Autodesk Fusion 360 part; units mm, degrees
(part 2 of 2)
sketch "スケッチ7 (3)" plane through (0, 0, 10.11) normal (0, 0, 1) x (1, 0, 0) in component "Robot V1 - B Front Cover"
  arc A0 (9.5, 66) -> (7.5, 68) centre (7.5, 66) ccw
  arc A1 (7.5, 56) -> (9.5, 58) centre (7.5, 58) ccw
  arc A2 (-16.5, 58) -> (-14.5, 56) centre (-14.5, 58) ccw
  arc A3 (-14.5, 68) -> (-16.5, 66) centre (-14.5, 66) ccw
  line L0 (-14.5, 68) -> (7.5, 68)
  line L1 (9.5, 66) -> (9.5, 58)
  line L2 (7.5, 56) -> (-14.5, 56)
  line L3 (-16.5, 58) -> (-16.5, 66)
  line L4 (7.5, 66) -> (-14.5, 58) construction
  point P0 (-3.5, 62)
  dimension "d1668" = 22
  dimension "d1669" = 8
  dimension "d1670" = 2
  dimension "d1671" = 3.5
  dimension "d1672" = 62
  constraint horizontal L0
  constraint horizontal L2
  constraint vertical L3
  constraint vertical L1
  constraint tangent A0 L0
  constraint tangent A0 L1
  constraint tangent A1 L1
  constraint tangent A1 L2
  constraint tangent A2 L2
  constraint tangent A2 L3
  constraint tangent A3 L3
  constraint tangent A3 L0
  constraint equal A0 A1
  constraint equal A0 A2
  constraint equal A0 A3
  constraint midpoint L4 P0
  measures "d1668" horizontal distance of A0.end A3.start
  measures "d1669" vertical distance of A0.start A1.end
  measures "d1670" radius of A0
  measures "d1671" horizontal distance of origin P0
  measures "d1672" vertical distance of origin P0
extrude "B07 Forehead opening" cut sketch "スケッチ7 (3)" against normal blind 2.4 bodies 18 in component "Robot V1 - B Front Cover"
sketch "スケッチ8 (3)" plane through (0, 0, 10.11) normal (0, 0, 1) x (1, 0, 0) in component "Robot V1 - B Front Cover"
  circle A0 centre (0, -59.97) radius 7
  dimension "d1675" = 59.97
  dimension "d1676" = 14
  constraint vertical origin A0.centre
  measures "d1675" vertical distance of origin A0.centre
  measures "d1676" diameter of A0
extrude "B08 Home access" cut sketch "スケッチ8 (3)" against normal blind 2.4 bodies 18 in component "Robot V1 - B Front Cover"
sketch "スケッチ9 (3)" plane through (0, 0, 10.11) normal (0, 0, 1) x (1, 0, 0) in component "Robot V1 - B Front Cover"
  line L0 (12, 16.1) -> (-12, 16.1)
  line L1 (-12, 16.1) -> (-12, 14.9)
  line L2 (-12, 14.9) -> (12, 14.9)
  line L3 (12, 14.9) -> (12, 16.1)
  line L4 (12, 16.1) -> (-12, 14.9) construction
  point P0 (0, 15.5)
  dimension "d1679" = 15.5
  dimension "d1680" = 24
  dimension "d1681" = 1.2
  constraint horizontal L0
  constraint vertical L1
  constraint horizontal L2
  constraint vertical L3
  constraint midpoint L4 P0
  constraint vertical origin P0
  measures "d1679" vertical distance of origin P0
  measures "d1680" horizontal distance of L0.start L0.end
  measures "d1681" vertical distance of L0.end L1.end
extrude "B09 Shallow mouth groove" cut sketch "スケッチ9 (3)" against normal blind 0.6 bodies 18 in component "Robot V1 - B Front Cover"
sketch "スケッチ19 (2)" plane through (0, 0, 7.71) normal (0, 0, 1) x (1, 0, 0) in component "Robot V1 - A Holder and Stand"
  circle A0 centre (-40, 62) radius 1.7
  dimension "d1684" = 40
  dimension "d1685" = 62
  dimension "d1686" = 3.4
  measures "d1684" horizontal distance of origin A0.centre
  measures "d1685" vertical distance of origin A0.centre
  measures "d1686" diameter of A0
extrude "A20 TL bolt hole" cut sketch "スケッチ19 (2)" against normal blind 10.61 bodies 17 in component "Robot V1 - A Holder and Stand"
sketch "スケッチ20" plane through (0, 0, 7.71) normal (0, 0, 1) x (1, 0, 0) in component "Robot V1 - A Holder and Stand"
  circle A0 centre (40, 62) radius 1.7
  dimension "d1689" = 40
  dimension "d1690" = 62
  dimension "d1691" = 3.4
  measures "d1689" horizontal distance of origin A0.centre
  measures "d1690" vertical distance of origin A0.centre
  measures "d1691" diameter of A0
extrude "A20 TR bolt hole" cut sketch "スケッチ20" against normal blind 10.61 bodies 17 in component "Robot V1 - A Holder and Stand"
sketch "スケッチ21" plane through (0, 0, 7.71) normal (0, 0, 1) x (1, 0, 0) in component "Robot V1 - A Holder and Stand"
  circle A0 centre (-37, -62) radius 1.7
  dimension "d1694" = 37
  dimension "d1695" = 62
  dimension "d1696" = 3.4
  measures "d1694" horizontal distance of origin A0.centre
  measures "d1695" vertical distance of origin A0.centre
  measures "d1696" diameter of A0
extrude "A20 BL bolt hole" cut sketch "スケッチ21" against normal blind 10.61 bodies 17 in component "Robot V1 - A Holder and Stand"
sketch "スケッチ22" plane through (0, 0, 7.71) normal (0, 0, 1) x (1, 0, 0) in component "Robot V1 - A Holder and Stand"
  circle A0 centre (37, -62) radius 1.7
  dimension "d1699" = 37
  dimension "d1700" = 62
  dimension "d1701" = 3.4
  measures "d1699" horizontal distance of origin A0.centre
  measures "d1700" vertical distance of origin A0.centre
  measures "d1701" diameter of A0
extrude "A20 BR bolt hole" cut sketch "スケッチ22" against normal blind 10.61 bodies 17 in component "Robot V1 - A Holder and Stand"
sketch "スケッチ10 (3)" plane through (0, 0, 10.11) normal (0, 0, 1) x (1, 0, 0) in component "Robot V1 - B Front Cover"
  circle A0 centre (-40, 62) radius 1.7
  dimension "d1704" = 40
  dimension "d1705" = 62
  dimension "d1706" = 3.4
  measures "d1704" horizontal distance of origin A0.centre
  measures "d1705" vertical distance of origin A0.centre
  measures "d1706" diameter of A0
extrude "B20 TL bolt hole" cut sketch "スケッチ10 (3)" against normal blind 2.4 bodies 18 in component "Robot V1 - B Front Cover"
sketch "スケッチ11 (3)" plane through (0, 0, 10.11) normal (0, 0, 1) x (1, 0, 0) in component "Robot V1 - B Front Cover"
  circle A0 centre (40, 62) radius 1.7
  dimension "d1709" = 40
  dimension "d1710" = 62
  dimension "d1711" = 3.4
  measures "d1709" horizontal distance of origin A0.centre
  measures "d1710" vertical distance of origin A0.centre
  measures "d1711" diameter of A0
extrude "B20 TR bolt hole" cut sketch "スケッチ11 (3)" against normal blind 2.4 bodies 18 in component "Robot V1 - B Front Cover"
sketch "スケッチ12 (3)" plane through (0, 0, 10.11) normal (0, 0, 1) x (1, 0, 0) in component "Robot V1 - B Front Cover"
  circle A0 centre (-37, -62) radius 1.7
  dimension "d1714" = 37
  dimension "d1715" = 62
  dimension "d1716" = 3.4
  measures "d1714" horizontal distance of origin A0.centre
  measures "d1715" vertical distance of origin A0.centre
  measures "d1716" diameter of A0
extrude "B20 BL bolt hole" cut sketch "スケッチ12 (3)" against normal blind 2.4 bodies 18 in component "Robot V1 - B Front Cover"
sketch "スケッチ13 (3)" plane through (0, 0, 10.11) normal (0, 0, 1) x (1, 0, 0) in component "Robot V1 - B Front Cover"
  circle A0 centre (37, -62) radius 1.7
  dimension "d1719" = 37
  dimension "d1720" = 62
  dimension "d1721" = 3.4
  measures "d1719" horizontal distance of origin A0.centre
  measures "d1720" vertical distance of origin A0.centre
  measures "d1721" diameter of A0
extrude "B20 BR bolt hole" cut sketch "スケッチ13 (3)" against normal blind 2.4 bodies 18 in component "Robot V1 - B Front Cover"
component "iPhone SE 3 - Parametric Drawing Model" placed x (1, 0, 0) y (0, 1, 0) z (0, 0, 1) at (0, 0, 0)
component "Robot V1 - A Holder and Stand" placed x (1, 0, 0) y (0, 1, 0) z (0, 0, 1) at (0, 0, 0)
component "Robot V1 - B Front Cover" placed x (1, 0, 0) y (0, 1, 0) z (0, 0, 1) at (0, 0, 0)
equation "SE3_OverallWidth = 67.27 mm" comment "Overall product width"
equation "SE3_OverallHeight = 138.44 mm" comment "Overall product height"
equation "SE3_ProductThickness = 7.31 mm" comment "Nominal product thickness"
equation "SE3_CornerRadius = 9.10 mm" comment "Parameterized plan-view corner radius"
equation "SE3_RearGlassThickness = 0.90 mm" comment "Modeled rear glass thickness"
equation "SE3_FrontGlassThickness = 0.90 mm" comment "Modeled front glass thickness"
equation "SE3_ActiveWidth = 58.50 mm" comment "Front active-area width"
equation "SE3_ActiveHeight = 104.05 mm" comment "Front active-area height"
equation "SE3_ActiveTopOffset = 17.19 mm" comment "Top product datum to active area"
equation "SE3_HomeDiameter = 10.90 mm" comment "Home/Touch ID sensor diameter"
equation "SE3_HomeBottomOffset = 9.25 mm" comment "Bottom datum to Home sensor center"
equation "SE3_ReceiverWidth = 11.87 mm" comment "Receiver width"
equation "SE3_ReceiverHeight = 1.20 mm" comment "Receiver height"
equation "SE3_ReceiverTopOffset = 9.10 mm" comment "Top datum to receiver center"
equation "SE3_FrontCameraDiameter = 3.21 mm" comment "Front camera opening/keepout diameter"
equation "SE3_FrontCameraXFromLeft = 22.99 mm" comment "Left datum to front camera center"
equation "SE3_FrontCameraTopOffset = 9.10 mm" comment "Top datum to front camera center"
equation "SE3_ProximityDiameter = 2.00 mm" comment "Proximity sensor display diameter"
equation "SE3_ProximityXFromLeft = 33.63 mm" comment "Left datum to proximity center"
equation "SE3_ProximityTopOffset = 4.84 mm" comment "Top datum to proximity center"
equation "SE3_ALSDiameter = 2.00 mm" comment "Ambient light sensor display diameter"
equation "SE3_ALSXFromLeft = 37.32 mm" comment "Left datum to ALS center"
equation "SE3_ALSTopOffset = 4.84 mm" comment "Top datum to ALS center"
equation "SE3_RearCameraDiameter = 8.57 mm" comment "Rear camera opening diameter"
equation "SE3_RearMicDiameter = 1.50 mm" comment "Rear microphone diameter"
equation "SE3_RearFlashDiameter = 3.75 mm" comment "Rear flash diameter"
equation "SE3_RearCameraXFromLeft = 10.44 mm" comment "Left datum to rear camera center"
equation "SE3_RearMicXFromLeft = 18.13 mm" comment "Left datum to rear microphone center"
equation "SE3_RearFlashXFromLeft = 22.84 mm" comment "Left datum to rear flash center"
equation "SE3_RearFeatureTopOffset = 15.40 mm" comment "Top datum to rear feature centers"
equation "SE3_CameraBumpHeight = 0.87 mm" comment "Modeled rear camera projection"
equation "SE3_RingTopOffset = 17.56 mm" comment "Top datum to top of ring/silent switch"
equation "SE3_RingLength = 5.61 mm" comment "Ring/silent switch length"
equation "SE3_VolumePlusCenterFromTop = 34.56 mm" comment "Top datum to volume-plus center"
equation "SE3_VolumeMinusCenterFromTop = 47.17 mm" comment "Top datum to volume-minus center"
equation "SE3_ButtonLength = 10.62 mm" comment "Button length: 2 x 5.31"
equation "SE3_ButtonFaceWidth = 1.80 mm" comment "Modeled button width in product-thickness direction"
equation "SE3_RingProjection = 0.42 mm" comment "Ring/silent switch projection"
equation "SE3_ButtonProjection = 0.40 mm" comment "Volume and side-button projection"
equation "SE3_SideButtonCenterFromTop = 34.64 mm" comment "Top datum to side-button center"
equation "SE3_SIMTrayTopOffset = 52.72 mm" comment "Top datum to SIM tray top"
equation "SE3_SIMTrayLength = 15.67 mm" comment "SIM tray length"
equation "SE3_SIMTrayWidth = 2.30 mm" comment "SIM tray visible width"
equation "SE3_BottomHoleDiameter = 1.45 mm" comment "Bottom microphone/speaker hole diameter"
equation "SE3_BottomHoleFirstFromLeft = 10.26 mm" comment "Left datum to first left acoustic hole"
equation "SE3_BottomHolePitch = 2.40 mm" comment "Bottom acoustic-hole pitch: 12.00 / 5"
equation "SE3_BottomRightFirstFromLeft = 45.01 mm" comment "Left datum to first right acoustic hole"
equation "SE3_ScrewDiameter = 1.60 mm" comment "Bottom screw diameter"
equation "SE3_LeftScrewFromLeft = 27.24 mm" comment "Left datum to left screw"
equation "SE3_RightScrewFromLeft = 40.03 mm" comment "Left datum to right screw"
equation "SE3_LightningWidth = 8.70 mm" comment "Lightning opening width: 37.98 - 29.28"
equation "SE3_LightningHeight = 1.60 mm" comment "Modeled Lightning opening height"
equation "SE3_DetailOverlay = 0.02 mm" comment "Visual reference overlay thickness"
equation "d710 = SE3_OverallWidth - 2 * SE3_CornerRadius"
equation "d711 = SE3_OverallHeight - 2 * SE3_CornerRadius"
equation "d712 = SE3_CornerRadius"
equation "d713 = SE3_OverallWidth / 2 - SE3_CornerRadius"
equation "d714 = SE3_OverallHeight / 2 - SE3_CornerRadius"
equation "d715 = SE3_RearGlassThickness"
equation "d717 = SE3_RearGlassThickness"
equation "d719 = SE3_OverallWidth - 2 * SE3_CornerRadius"
equation "d720 = SE3_OverallHeight - 2 * SE3_CornerRadius"
equation "d721 = SE3_CornerRadius"
equation "d722 = SE3_OverallWidth / 2 - SE3_CornerRadius"
equation "d723 = SE3_OverallHeight / 2 - SE3_CornerRadius"
equation "d724 = SE3_ProductThickness - SE3_RearGlassThickness - SE3_FrontGlassThickness"
equation "d726 = SE3_ProductThickness - SE3_FrontGlassThickness"
equation "d728 = SE3_OverallWidth - 2 * SE3_CornerRadius"
equation "d729 = SE3_OverallHeight - 2 * SE3_CornerRadius"
equation "d730 = SE3_CornerRadius"
equation "d731 = SE3_OverallWidth / 2 - SE3_CornerRadius"
equation "d732 = SE3_OverallHeight / 2 - SE3_CornerRadius"
equation "d733 = SE3_FrontGlassThickness"
equation "d735 = SE3_ProductThickness"
equation "d737 = SE3_ActiveWidth - 2 * 0.80 mm"
equation "d738 = SE3_ActiveHeight - 2 * 0.80 mm"
equation "d740 = SE3_ActiveWidth / 2 - 0.80 mm"
equation "d741 = ( SE3_OverallHeight / 2 - SE3_ActiveTopOffset - SE3_ActiveHeight / 2 ) + SE3_ActiveHeight / 2 - 0.80 mm"
equation "d742 = SE3_DetailOverlay"
equation "d744 = SE3_OverallHeight / 2 - SE3_HomeBottomOffset"
equation "d745 = SE3_HomeDiameter"
equation "d746 = SE3_DetailOverlay"
equation "d748 = SE3_OverallWidth / 2 - SE3_FrontCameraXFromLeft"
equation "d749 = SE3_OverallHeight / 2 - SE3_FrontCameraTopOffset"
equation "d750 = SE3_FrontCameraDiameter"
equation "d751 = SE3_DetailOverlay"
equation "d753 = SE3_OverallWidth / 2 - SE3_ProximityXFromLeft"
equation "d754 = SE3_OverallHeight / 2 - SE3_ProximityTopOffset"
equation "d755 = SE3_ProximityDiameter"
equation "d756 = SE3_DetailOverlay"
equation "d758 = SE3_ALSXFromLeft - SE3_OverallWidth / 2"
equation "d759 = SE3_OverallHeight / 2 - SE3_ALSTopOffset"
equation "d760 = SE3_ALSDiameter"
equation "d761 = SE3_DetailOverlay"
equation "d763 = SE3_ReceiverWidth - SE3_ReceiverHeight"
equation "d764 = SE3_ReceiverHeight / 2"
equation "d765 = SE3_OverallHeight / 2 - SE3_ReceiverTopOffset"
equation "d766 = SE3_DetailOverlay"
equation "d768 = SE3_OverallWidth / 2 - SE3_RearCameraXFromLeft"
equation "d769 = SE3_OverallHeight / 2 - SE3_RearFeatureTopOffset"
equation "d770 = SE3_RearCameraDiameter"
equation "d771 = -( SE3_CameraBumpHeight )"
equation "d773 = SE3_OverallWidth / 2 - SE3_RearMicXFromLeft"
equation "d774 = SE3_OverallHeight / 2 - SE3_RearFeatureTopOffset"
equation "d775 = SE3_RearMicDiameter"
equation "d776 = -( SE3_DetailOverlay )"
equation "d778 = SE3_OverallWidth / 2 - SE3_RearFlashXFromLeft"
equation "d779 = SE3_OverallHeight / 2 - SE3_RearFeatureTopOffset"
equation "d780 = SE3_RearFlashDiameter"
equation "d781 = -( SE3_DetailOverlay )"
equation "d783 = -SE3_OverallWidth / 2"
equation "d785 = SE3_OverallWidth / 2"
equation "d787 = SE3_RingLength - SE3_ButtonFaceWidth"
equation "d788 = SE3_ButtonFaceWidth / 2"
equation "d789 = SE3_ProductThickness / 2"
equation "d790 = SE3_OverallHeight / 2 - SE3_RingTopOffset - SE3_RingLength / 2"
equation "d791 = -( SE3_RingProjection )"
equation "d793 = SE3_ButtonLength - SE3_ButtonFaceWidth"
equation "d794 = SE3_ButtonFaceWidth / 2"
equation "d795 = SE3_ProductThickness / 2"
equation "d796 = SE3_OverallHeight / 2 - SE3_VolumePlusCenterFromTop"
equation "d797 = -( SE3_ButtonProjection )"
equation "d799 = SE3_ButtonLength - SE3_ButtonFaceWidth"
equation "d800 = SE3_ButtonFaceWidth / 2"
equation "d801 = SE3_ProductThickness / 2"
equation "d802 = SE3_OverallHeight / 2 - SE3_VolumeMinusCenterFromTop"
equation "d803 = -( SE3_ButtonProjection )"
equation "d805 = SE3_ButtonLength - SE3_ButtonFaceWidth"
equation "d806 = SE3_ButtonFaceWidth / 2"
equation "d807 = SE3_ProductThickness / 2"
equation "d808 = SE3_OverallHeight / 2 - SE3_SideButtonCenterFromTop"
equation "d809 = SE3_ButtonProjection"
equation "d811 = SE3_SIMTrayLength - SE3_SIMTrayWidth"
equation "d812 = SE3_SIMTrayWidth / 2"
equation "d813 = SE3_ProductThickness / 2"
equation "d814 = SE3_OverallHeight / 2 - SE3_SIMTrayTopOffset - SE3_SIMTrayLength / 2"
equation "d815 = -( 0.05 mm )"
equation "d817 = -SE3_OverallHeight / 2"
equation "d819 = SE3_LightningWidth - SE3_LightningHeight"
equation "d820 = SE3_LightningHeight / 2"
equation "d821 = SE3_ProductThickness / 2"
equation "d822 = SE3_OverallWidth / 2 - ( SE3_BottomHoleFirstFromLeft + 0 * SE3_BottomHolePitch )"
equation "d823 = SE3_ProductThickness / 2"
equation "d824 = SE3_BottomHoleDiameter"
equation "d825 = SE3_OverallWidth / 2 - ( SE3_BottomHoleFirstFromLeft + 1 * SE3_BottomHolePitch )"
equation "d826 = SE3_ProductThickness / 2"
equation "d827 = SE3_BottomHoleDiameter"
equation "d828 = SE3_OverallWidth / 2 - ( SE3_BottomHoleFirstFromLeft + 2 * SE3_BottomHolePitch )"
equation "d829 = SE3_ProductThickness / 2"
equation "d830 = SE3_BottomHoleDiameter"
equation "d831 = SE3_OverallWidth / 2 - ( SE3_BottomHoleFirstFromLeft + 3 * SE3_BottomHolePitch )"
equation "d832 = SE3_ProductThickness / 2"
equation "d833 = SE3_BottomHoleDiameter"
equation "d834 = SE3_OverallWidth / 2 - ( SE3_BottomHoleFirstFromLeft + 4 * SE3_BottomHolePitch )"
equation "d835 = SE3_ProductThickness / 2"
equation "d836 = SE3_BottomHoleDiameter"
equation "d837 = SE3_OverallWidth / 2 - ( SE3_BottomHoleFirstFromLeft + 5 * SE3_BottomHolePitch )"
equation "d838 = SE3_ProductThickness / 2"
equation "d839 = SE3_BottomHoleDiameter"
equation "d840 = ( SE3_BottomRightFirstFromLeft + 0 * SE3_BottomHolePitch ) - SE3_OverallWidth / 2"
equation "d841 = SE3_ProductThickness / 2"
equation "d842 = SE3_BottomHoleDiameter"
equation "d843 = ( SE3_BottomRightFirstFromLeft + 1 * SE3_BottomHolePitch ) - SE3_OverallWidth / 2"
equation "d844 = SE3_ProductThickness / 2"
equation "d845 = SE3_BottomHoleDiameter"
equation "d846 = ( SE3_BottomRightFirstFromLeft + 2 * SE3_BottomHolePitch ) - SE3_OverallWidth / 2"
equation "d847 = SE3_ProductThickness / 2"
equation "d848 = SE3_BottomHoleDiameter"
equation "d849 = ( SE3_BottomRightFirstFromLeft + 3 * SE3_BottomHolePitch ) - SE3_OverallWidth / 2"
equation "d850 = SE3_ProductThickness / 2"
equation "d851 = SE3_BottomHoleDiameter"
equation "d852 = ( SE3_BottomRightFirstFromLeft + 4 * SE3_BottomHolePitch ) - SE3_OverallWidth / 2"
equation "d853 = SE3_ProductThickness / 2"
equation "d854 = SE3_BottomHoleDiameter"
equation "d855 = ( SE3_BottomRightFirstFromLeft + 5 * SE3_BottomHolePitch ) - SE3_OverallWidth / 2"
equation "d856 = SE3_ProductThickness / 2"
equation "d857 = SE3_BottomHoleDiameter"
equation "d858 = SE3_OverallWidth / 2 - SE3_LeftScrewFromLeft"
equation "d859 = SE3_ProductThickness / 2"
equation "d860 = SE3_ScrewDiameter"
equation "d861 = SE3_RightScrewFromLeft - SE3_OverallWidth / 2"
equation "d862 = SE3_ProductThickness / 2"
equation "d863 = SE3_ScrewDiameter"
equation "d866 = SE3_ProductThickness / 2"
equation "d868 = SE3_OverallWidth - 2 * SE3_CornerRadius"
equation "d869 = SE3_OverallHeight - 2 * SE3_CornerRadius"
equation "d870 = SE3_CornerRadius"
equation "d871 = SE3_OverallWidth / 2 - SE3_CornerRadius"
equation "d872 = SE3_OverallHeight / 2 - SE3_CornerRadius"
equation "RB_Clearance = 0.4 mm" comment "Phone clearance PER SIDE; test-print before final use"
equation "RB_BackGap = 0.5 mm" comment "Allowance for thin pads between rear glass and tray"
equation "RB_FrontGap = 0.4 mm" comment "Clearance above front glass, excluding screen protector"
equation "RB_Wall = 2.4 mm" comment "Tray side walls"
equation "RB_BackThickness = 2.4 mm" comment "Tray back plate"
equation "RB_CoverThickness = 2.4 mm" comment "Front cover plate"
equation "RB_HeadWidth = 92 mm" comment "Head width, excluding no separate ears"
equation "RB_BodyWidth = 82 mm" comment "Body widened from concept to fit lower M3 screws"
equation "RB_CaseHeight = 148 mm" comment "Cover total height in phone coordinates"
equation "RB_HeadHeight = 60 mm" comment "Top rounded box height"
equation "RB_BodyHeight = 96 mm" comment "Bottom rounded box height; overlaps head"
equation "RB_OuterRadius = 6 mm" comment "Rounded external corners"
equation "RB_EyeWidth = 20 mm" comment "Each eye aperture width"
equation "RB_EyeHeight = 22 mm" comment "Each eye aperture height"
equation "RB_EyeRadius = 8 mm" comment "Eye corner radius, <= half the smaller dimension"
equation "RB_EyeX = 14 mm" comment "Half of eye center spacing"
equation "RB_EyeY = 31 mm" comment "Eye centers above phone center"
equation "RB_BellyWidth = 48 mm" comment "Message window width"
equation "RB_BellyHeight = 28 mm" comment "Message window height"
equation "RB_BellyRadius = 3 mm" comment "Message window corner radius"
equation "RB_BellyY = -3 mm" comment "Message window center Y"
equation "RB_TalkDiameter = 24 mm" comment "Touch aperture at the screen side"
equation "RB_TalkY = -35 mm" comment "Touch aperture center Y"
equation "RB_TouchBevel = 1 mm" comment "45 degree entry bevel; remaining lip is 1.4 mm"
equation "RB_HomeDiameter = 14 mm" comment "Maintenance access, NOT the conversation button"
equation "RB_ForeheadWidth = 26 mm" comment "Camera, receiver, sensors shared forehead opening"
equation "RB_ForeheadHeight = 12 mm" comment "Forehead opening; validate camera field of view"
equation "RB_ForeheadX = -3.5 mm" comment "Forehead opening center X"
equation "RB_ForeheadY = 62 mm" comment "Forehead opening center Y"
equation "RB_MouthWidth = 24 mm" comment "Decorative mouth groove width"
equation "RB_MouthHeight = 1.2 mm" comment "Decorative mouth groove height"
equation "RB_MouthY = 15.5 mm" comment "Decorative mouth center Y"
equation "RB_MouthDepth = 0.6 mm" comment "Blind groove only, no display opening"
equation "RB_ScrewDiameter = 3.4 mm" comment "Through clearance for four M3 bolts and loose nuts"
equation "RB_TopScrewX = 40 mm" comment "Top screw centers +/- X"
equation "RB_TopScrewY = 62 mm" comment "Top screw centers Y"
equation "RB_BottomScrewX = 37 mm" comment "Bottom screw centers +/- X"
equation "RB_BottomScrewY = -62 mm" comment "Bottom screw centers Y"
equation "RB_Tilt = 12 deg" comment "Phone tilt back from vertical on its base"
equation "RB_Lift = 35 mm" comment "Desk to phone lower rear edge; check actual cable"
equation "RB_BaseWidth = 100 mm" comment "Base left-right width"
equation "RB_BaseDepth = 90 mm" comment "Base front-back distance along desk"
equation "RB_BaseFront = 20 mm" comment "Base reach forward from lower rear-edge projection"
equation "RB_BaseThickness = 4 mm" comment "Base thickness normal to desk"
equation "RB_RibThickness = 4 mm" comment "Two rear triangular stand ribs"
equation "RB_RibX = 29 mm" comment "Stand rib center X +/-"
equation "RB_CableWidth = 16 mm" comment "Open-ended cable channel in base"
equation "RB_BottomOpening = 54 mm" comment "Bottom opening clears Lightning and both acoustic rows"
equation "RB_VentWidth = 40 mm" comment "Rear ventilation / finger access width"
equation "RB_VentHeight = 62 mm" comment "Rear ventilation / finger access height"
equation "RB_RearCameraWidth = 26 mm" comment "Rear camera, microphone and flash opening"
equation "RB_RearCameraHeight = 18 mm" comment "Rear camera opening height"
equation "RB_PocketWidth = SE3_OverallWidth + 2 * RB_Clearance" comment "Derived phone pocket width"
equation "RB_PocketHeight = SE3_OverallHeight + 2 * RB_Clearance" comment "Derived phone pocket height"
equation "RB_PocketRadius = SE3_CornerRadius + RB_Clearance" comment "Derived approximate pocket corner radius"
equation "RB_TrayWidth = RB_PocketWidth + 2 * RB_Wall" comment "Derived outer tray width"
equation "RB_TrayHeight = RB_PocketHeight + 2 * RB_Wall" comment "Derived outer tray height"
equation "RB_BackZ = -RB_BackGap - RB_BackThickness" comment "Rear-most tray plane"
equation "RB_CoverZ = SE3_ProductThickness + RB_FrontGap" comment "Cover rear face / tray mating plane"
equation "RB_CoverTopZ = RB_CoverZ + RB_CoverThickness" comment "Cover front face"
equation "RB_DeskY = -SE3_OverallHeight / 2 - RB_Lift / cos(RB_Tilt)" comment "Desk-plane Y intercept at phone Z=0"
equation "d1514 = RB_BackZ"
equation "d1516 = -RB_BackGap"
equation "d1518 = RB_CoverZ"
equation "d1520 = ( RB_HeadWidth ) - 2 * ( RB_OuterRadius )"
equation "d1521 = ( RB_HeadHeight ) - 2 * ( RB_OuterRadius )"
equation "d1522 = RB_OuterRadius"
equation "d1523 = abs(RB_CaseHeight / 2 - RB_HeadHeight / 2)"
equation "d1524 = RB_BackThickness"
equation "d1526 = ( RB_BodyWidth ) - 2 * ( RB_OuterRadius )"
equation "d1527 = ( RB_BodyHeight ) - 2 * ( RB_OuterRadius )"
equation "d1528 = RB_OuterRadius"
equation "d1529 = abs(-RB_CaseHeight / 2 + RB_BodyHeight / 2)"
equation "d1530 = RB_BackThickness"
equation "d1532 = ( RB_TrayWidth ) - 2 * ( RB_PocketRadius + RB_Wall )"
equation "d1533 = ( RB_TrayHeight ) - 2 * ( RB_PocketRadius + RB_Wall )"
equation "d1534 = RB_PocketRadius + RB_Wall"
equation "d1535 = RB_CoverZ + RB_BackGap"
equation "d1537 = abs(-RB_TopScrewX)"
equation "d1538 = abs(RB_TopScrewY)"
equation "d1540 = RB_CoverZ + RB_BackGap"
equation "d1542 = abs(RB_TopScrewX)"
equation "d1543 = abs(RB_TopScrewY)"
equation "d1545 = RB_CoverZ + RB_BackGap"
equation "d1547 = abs(-RB_BottomScrewX)"
equation "d1548 = abs(RB_BottomScrewY)"
equation "d1550 = RB_CoverZ + RB_BackGap"
equation "d1552 = abs(RB_BottomScrewX)"
equation "d1553 = abs(RB_BottomScrewY)"
equation "d1555 = RB_CoverZ + RB_BackGap"
equation "d1557 = ( RB_PocketWidth ) - 2 * ( RB_PocketRadius )"
equation "d1558 = ( RB_PocketHeight ) - 2 * ( RB_PocketRadius )"
equation "d1559 = RB_PocketRadius"
equation "d1560 = -( RB_CoverZ + RB_BackGap )"
equation "d1562 = abs(-RB_TrayWidth / 2)"
equation "d1563 = abs(34 mm)"
equation "d1566 = -( RB_CoverZ + RB_BackGap )"
equation "d1568 = abs(RB_TrayWidth / 2)"
equation "d1569 = abs(34 mm)"
equation "d1572 = -( RB_CoverZ + RB_BackGap )"
equation "d1574 = abs(-RB_CaseHeight / 2)"
equation "d1575 = RB_BottomOpening"
equation "d1577 = -( RB_CoverZ - RB_BackZ )"
equation "d1579 = ( RB_RearCameraWidth ) - 2 * ( 2 mm )"
equation "d1580 = ( RB_RearCameraHeight ) - 2 * ( 2 mm )"
equation "d1582 = abs(-18 mm)"
equation "d1583 = abs(54.5 mm)"
equation "d1584 = -( RB_CoverZ - RB_BackZ )"
equation "d1586 = ( RB_VentWidth ) - 2 * ( 4 mm )"
equation "d1587 = ( RB_VentHeight ) - 2 * ( 4 mm )"
equation "d1589 = abs(-7 mm)"
equation "d1590 = -( RB_CoverZ - RB_BackZ )"
equation "d1592 = -RB_RibX - RB_RibThickness / 2"
equation "d1594 = abs(( -1 ) * ( -RB_BackGap ))"
equation "d1595 = abs(RB_DeskY - ( -RB_BackGap ) * tan(RB_Tilt) + RB_BaseThickness / cos(RB_Tilt) - 0.3 mm)"
equation "d1596 = abs(( -1 ) * ( -( RB_BaseDepth - RB_BaseFront - 4 mm ) * cos(RB_Tilt) ))"
equation "d1597 = abs(RB_DeskY - ( -( RB_BaseDepth - RB_BaseFront - 4 mm ) * cos(RB_Tilt) ) * tan(RB_Tilt) + RB_BaseThickness / cos(RB_Tilt) - 0.3 mm)"
equation "d1598 = RB_RibThickness"
equation "d1600 = RB_RibX - RB_RibThickness / 2"
equation "d1602 = abs(( -1 ) * ( -RB_BackGap ))"
equation "d1603 = abs(RB_DeskY - ( -RB_BackGap ) * tan(RB_Tilt) + RB_BaseThickness / cos(RB_Tilt) - 0.3 mm)"
equation "d1604 = abs(( -1 ) * ( -( RB_BaseDepth - RB_BaseFront - 4 mm ) * cos(RB_Tilt) ))"
equation "d1605 = abs(RB_DeskY - ( -( RB_BaseDepth - RB_BaseFront - 4 mm ) * cos(RB_Tilt) ) * tan(RB_Tilt) + RB_BaseThickness / cos(RB_Tilt) - 0.3 mm)"
equation "d1606 = RB_RibThickness"
equation "d1608 = -RB_BaseWidth / 2"
equation "d1610 = abs(( -1 ) * ( RB_BaseFront * cos(RB_Tilt) ))"
equation "d1611 = abs(RB_DeskY - ( RB_BaseFront * cos(RB_Tilt) ) * tan(RB_Tilt))"
equation "d1612 = abs(( -1 ) * ( -( RB_BaseDepth - RB_BaseFront ) * cos(RB_Tilt) ))"
equation "d1613 = abs(RB_DeskY - ( -( RB_BaseDepth - RB_BaseFront ) * cos(RB_Tilt) ) * tan(RB_Tilt))"
equation "d1614 = abs(( -1 ) * ( ( -( RB_BaseDepth - RB_BaseFront ) * cos(RB_Tilt) ) + RB_BaseThickness * sin(RB_Tilt) ))"
equation "d1615 = abs(RB_DeskY - ( ( -( RB_BaseDepth - RB_BaseFront ) * cos(RB_Tilt) ) + RB_BaseThickness * sin(RB_Tilt) ) * tan(RB_Tilt) + RB_BaseThickness / cos(RB_Tilt))"
equation "d1616 = abs(( -1 ) * ( ( RB_BaseFront * cos(RB_Tilt) ) + RB_BaseThickness * sin(RB_Tilt) ))"
equation "d1617 = abs(RB_DeskY - ( ( RB_BaseFront * cos(RB_Tilt) ) + RB_BaseThickness * sin(RB_Tilt) ) * tan(RB_Tilt) + RB_BaseThickness / cos(RB_Tilt))"
equation "d1618 = RB_BaseWidth"
equation "d1622 = abs(RB_DeskY)"
equation "d1623 = RB_CableWidth"
equation "d1624 = RB_BaseDepth"
equation "d1625 = -RB_BaseDepth"
equation "d1627 = RB_CoverZ"
equation "d1629 = RB_CoverTopZ"
equation "d1631 = ( RB_HeadWidth ) - 2 * ( RB_OuterRadius )"
equation "d1632 = ( RB_HeadHeight ) - 2 * ( RB_OuterRadius )"
equation "d1633 = RB_OuterRadius"
equation "d1634 = abs(RB_CaseHeight / 2 - RB_HeadHeight / 2)"
equation "d1635 = RB_CoverThickness"
equation "d1637 = ( RB_BodyWidth ) - 2 * ( RB_OuterRadius )"
equation "d1638 = ( RB_BodyHeight ) - 2 * ( RB_OuterRadius )"
equation "d1639 = RB_OuterRadius"
equation "d1640 = abs(-RB_CaseHeight / 2 + RB_BodyHeight / 2)"
equation "d1641 = RB_CoverThickness"
equation "d1643 = ( RB_EyeWidth ) - 2 * ( RB_EyeRadius )"
equation "d1644 = ( RB_EyeHeight ) - 2 * ( RB_EyeRadius )"
equation "d1645 = RB_EyeRadius"
equation "d1646 = abs(-RB_EyeX)"
equation "d1647 = abs(RB_EyeY)"
equation "d1648 = -RB_CoverThickness"
equation "d1650 = ( RB_EyeWidth ) - 2 * ( RB_EyeRadius )"
equation "d1651 = ( RB_EyeHeight ) - 2 * ( RB_EyeRadius )"
equation "d1652 = RB_EyeRadius"
equation "d1653 = abs(RB_EyeX)"
equation "d1654 = abs(RB_EyeY)"
equation "d1655 = -RB_CoverThickness"
equation "d1657 = ( RB_BellyWidth ) - 2 * ( RB_BellyRadius )"
equation "d1658 = ( RB_BellyHeight ) - 2 * ( RB_BellyRadius )"
equation "d1659 = RB_BellyRadius"
equation "d1660 = abs(RB_BellyY)"
equation "d1661 = -RB_CoverThickness"
equation "d1663 = abs(RB_TalkY)"
equation "d1664 = RB_TalkDiameter"
equation "d1665 = -RB_CoverThickness"
equation "d1667 = RB_TouchBevel"
equation "d1668 = ( RB_ForeheadWidth ) - 2 * ( 2 mm )"
equation "d1669 = ( RB_ForeheadHeight ) - 2 * ( 2 mm )"
equation "d1671 = abs(RB_ForeheadX)"
equation "d1672 = abs(RB_ForeheadY)"
equation "d1673 = -RB_CoverThickness"
equation "d1675 = abs(-SE3_OverallHeight / 2 + SE3_HomeBottomOffset)"
equation "d1676 = RB_HomeDiameter"
equation "d1677 = -RB_CoverThickness"
equation "d1679 = abs(RB_MouthY)"
equation "d1680 = RB_MouthWidth"
equation "d1681 = RB_MouthHeight"
equation "d1682 = -RB_MouthDepth"
equation "d1684 = abs(-RB_TopScrewX)"
equation "d1685 = abs(RB_TopScrewY)"
equation "d1686 = RB_ScrewDiameter"
equation "d1687 = -( RB_CoverZ - RB_BackZ )"
equation "d1689 = abs(RB_TopScrewX)"
equation "d1690 = abs(RB_TopScrewY)"
equation "d1691 = RB_ScrewDiameter"
equation "d1692 = -( RB_CoverZ - RB_BackZ )"
equation "d1694 = abs(-RB_BottomScrewX)"
equation "d1695 = abs(RB_BottomScrewY)"
equation "d1696 = RB_ScrewDiameter"
equation "d1697 = -( RB_CoverZ - RB_BackZ )"
equation "d1699 = abs(RB_BottomScrewX)"
equation "d1700 = abs(RB_BottomScrewY)"
equation "d1701 = RB_ScrewDiameter"
equation "d1702 = -( RB_CoverZ - RB_BackZ )"
equation "d1704 = abs(-RB_TopScrewX)"
equation "d1705 = abs(RB_TopScrewY)"
equation "d1706 = RB_ScrewDiameter"
equation "d1707 = -RB_CoverThickness"
equation "d1709 = abs(RB_TopScrewX)"
equation "d1710 = abs(RB_TopScrewY)"
equation "d1711 = RB_ScrewDiameter"
equation "d1712 = -RB_CoverThickness"
equation "d1714 = abs(-RB_BottomScrewX)"
equation "d1715 = abs(RB_BottomScrewY)"
equation "d1716 = RB_ScrewDiameter"
equation "d1717 = -RB_CoverThickness"
equation "d1719 = abs(RB_BottomScrewX)"
equation "d1720 = abs(RB_BottomScrewY)"
equation "d1721 = RB_ScrewDiameter"
equation "d1722 = -RB_CoverThickness"
named bodies: "Rear Glass", "Aluminum Frame", "Front Cover Glass", "Front Active Area Reference", "Home Touch ID Sensor", "Front Detail 12 Front Camera Position", "Front Detail 13 Proximity Sensor Position", "Front Detail 14 ALS Position", "Receiver Opening", "Rear Camera Bump", "Rear Microphone", "Rear Flash", "Ring Silent Switch", "Volume Plus Button", "Volume Minus Button", "Side Button", "A - White PLA holder and stand", "B - White PLA front cover"
